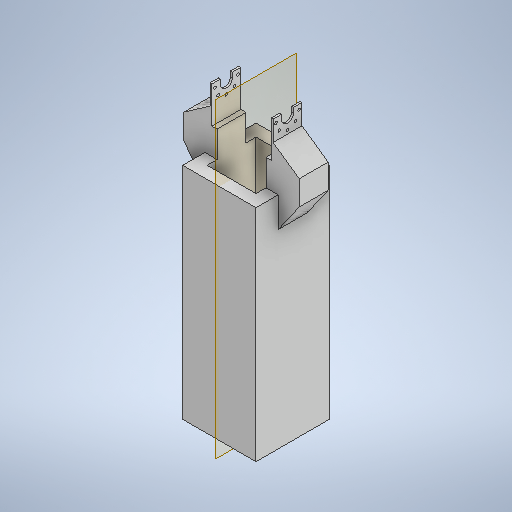
# Autodesk Inventor part: BiggerBracket
Saved by Autodesk Inventor 2027 (Build 310192060, 192F)
## iProperties
Created: 2026-07-12
Part Number: BiggerBracket
Material: Generic
Document SubType Name: Modeling
Designer: 13129
Density: 1 g/cm^3
Appearance: Default
Author: 13129
Autodesk Inventor part; units mm, degrees
ref_plane "XZ Plane" through (0, 0, 0) normal (0, 1, 0) x (-1, 0, 0)
ref_plane "XY Plane" through (0, 0, 0) normal (0, 0, 1) x (1, 0, 0)
sketch "Sketch1" plane through (0, 0, 0) normal (0, 1, 0) x (-1, 0, 0)
  line L0 (30.75, -15) -> (-30.75, -15)
  line L1 (-30.75, -15) -> (-30.75, 15)
  line L2 (-30.75, 15) -> (30.75, 15)
  line L3 (30.75, 15) -> (30.75, -15)
  point P0 (0, 0)
  point P1 (-30.75, 0)
  point P2 (0, -15)
  dimension "d0" = 61.5
  dimension "d1" = 30
  constraints: 8 end point, 3 perpendicular, 2 midpoint, 1 horizontal, 1 horizontal alignment, 1 vertical alignment
  measures "d0" distance of L0.start L0.end
  measures "d1" distance of L0.end L1.end
extrude "Extrusion1" add sketch "Sketch1" along normal blind 2
sketch "Sketch2" plane through (30.75, 0, 15) normal (1, 0, 0) x (0, 0, -1)
  line L0 (0, 0) -> (30, 0) construction
  line L1 (0, 2) -> (30, 2) construction
  line L2 (0, 0) -> (0, 40)
  line L3 (30, 0) -> (30, 40)
  line L4 (0, 0) -> (30, 0)
  circle A0 centre (15, 35) radius 12 construction
  arc A1 (8.75, 35) -> (21.25, 35) centre (15, 35) ccw
  line L5 (8.75, 40) -> (8.75, 35)
  line L6 (21.25, 40) -> (21.25, 35)
  line L7 (0, 40) -> (8.75, 40)
  line L8 (21.25, 40) -> (30, 40)
  circle A2 centre (3, 35) radius 1.4
  circle A3 centre (6.5147, 26.5147) radius 1.4
  circle A4 centre (15, 23) radius 1.4
  circle A5 centre (23.4853, 26.5147) radius 1.4
  circle A6 centre (27, 35) radius 1.4
  point P0 (15, 0)
  point P1 (15, 2)
  point P2 (15, 28.75)
  dimension "d5" = 24
  dimension "d4" = 40
  dimension "d6" = 35
  dimension "d7" = 12.5
  dimension "d9" = 2.8
  dimension "d12" = 180
  constraints: 14 end point, 6 centre point, 4 vertical, 3 horizontal alignment, 3 point on circle, 2 parallel, 2 tangent, 1 coincident, 1 collinear, 1 horizontal, 1 midpoint, 1 perpendicular, 1 vertical alignment, 11 other
  measures "d4" distance of L0.start L2.end
  measures "d6" vertical distance of L0.start point (15, 35)
  measures "d7" diameter of A1
  measures "d9" diameter of A2
extrude "Extrusion2" add sketch "Sketch2" along normal blind 2
mirror "Mirror1" about plane through (0, 0, 0) normal (1, 0, 0) of "Extrusion2"
sketch "Sketch3" plane through (30.75, 2, 15) normal (0, 0, 1) x (1, 0, 0)
  line L0 (-63.5, 38) -> (-63.5, -2) construction
  line L1 (-63.5, 17.05) -> (-90.7062, -2)
  line L2 (-63.5, 17.05) -> (-63.5, -2)
  line L3 (-63.5, -2) -> (-90.7062, -2)
  point P0 (-30.75, -2)
  dimension "d16" = 19.05
  dimension "d17" = 55
  constraints: 6 end point, 1 collinear, 1 perpendicular, 1 point on line
  measures "d16" distance of L0.end L1.start
  measures "d17" angle of L1 L0
extrude "Extrusion3" add sketch "Sketch3" against normal blind 30
mirror "Mirror2" about plane through (0, 0, 0) normal (1, 0, 0) of "Extrusion3"
sketch "Sketch4" plane through (0, 0, 0) normal (0, -1, 0) x (1, 0, 0)
  line L0 (-59.9562, 15) -> (59.9562, 15)
  line L1 (59.9562, 15) -> (59.9562, -15)
  line L2 (59.9562, -15) -> (-59.9562, -15)
  line L3 (-59.9562, -15) -> (-59.9562, 15)
  point P0 (0, 0)
  constraints: 8 end point, 2 parallel, 1 horizontal, 1 perpendicular
extrude "Extrusion4" add sketch "Sketch4" along normal blind 25.4
sketch "Sketch5" plane through (0, -25.4, 0) normal (0, -1, 0) x (1, 0, 0)
  line L0 (-38.1, 38.1) -> (38.1, 38.1)
  line L1 (38.1, 38.1) -> (38.1, -38.1)
  line L2 (38.1, -38.1) -> (-38.1, -38.1)
  line L3 (-38.1, -38.1) -> (-38.1, 38.1)
  point P0 (0, 0)
  point P1 (0, 38.1)
  point P2 (38.1, 0)
  dimension "d22" = 76.2
  dimension "d23" = 76.2
  constraints: 8 end point, 2 midpoint, 2 parallel, 1 horizontal, 1 horizontal alignment, 1 perpendicular, 1 vertical alignment
  measures "d22" distance of L1.end L2.end
  measures "d23" distance of L0.end L1.end
extrude "Extrusion5" add sketch "Sketch5" along normal blind 228.6
sketch "Sketch6" plane through (30.75, 2, 15) normal (0, 0, 1) x (1, 0, 0)
  line L0 (-90.7062, -27.4) -> (-68.85, -58.6139)
  line L1 (-68.85, -27.4) -> (-68.85, -256) construction
  line L2 (-90.7062, -27.4) -> (-52.6011, -27.4) construction
  line L3 (-90.7062, -27.4) -> (-68.85, -27.4)
  line L4 (-68.85, -58.6139) -> (-68.85, -27.4)
  point P0 (-30.75, -2)
  dimension "d26" = 55
  constraints: 8 end point, 2 collinear, 1 equal length, 1 horizontal, 1 point on line
  measures "d26" angle of L0 L2
extrude "Extrusion6" add sketch "Sketch6" against normal blind 30
mirror "Mirror3" about plane through (0, 0, 0) normal (1, 0, 0) of "Extrusion6"
sketch "Sketch7" plane through (0, -254, 0) normal (0, -1, 0) x (1, 0, 0)
  line L0 (38.1, -38.1) -> (38.1, 38.1) construction
  line L1 (38.1, 38.1) -> (-38.1, 38.1) construction
  line L2 (25.4, -25.4) -> (-25.4, -25.4)
  line L3 (-25.4, -25.4) -> (-25.4, 25.4)
  line L4 (-25.4, 25.4) -> (25.4, 25.4)
  line L5 (25.4, 25.4) -> (25.4, -25.4)
  point P0 (0, 0)
  point P1 (0, 25.4)
  point P2 (0, 38.1)
  point P3 (25.4, 0)
  point P4 (38.1, 0)
  dimension "d29" = 50.8
  dimension "d30" = 50.8
  constraints: 8 end point, 4 midpoint, 2 parallel, 1 horizontal, 1 horizontal alignment, 1 perpendicular, 1 vertical alignment
  measures "d29" distance of L3.end L4.end
  measures "d30" distance of L2.end L3.end
extrude "Extrusion7" cut sketch "Sketch7" against normal blind 260.1875
body "Solid1"
